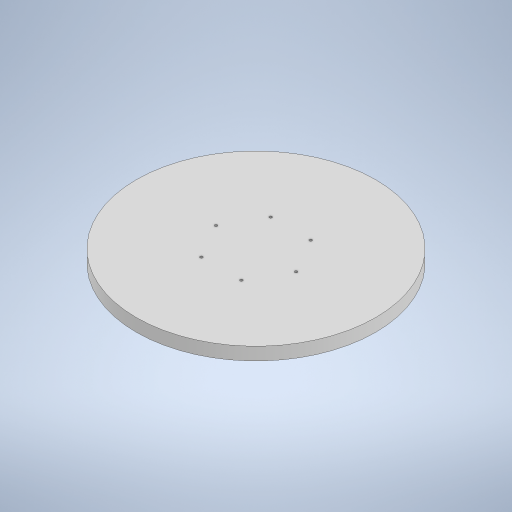
# Autodesk Inventor part: Lazy suzan Top piece
Saved by Autodesk Inventor 2023 (Build 270158000, 158)
## iProperties
Created: 2022-11-23
Part Number: Lazy suzan Top piece
Material: Generic
Document SubType Name: Modeling
Designer: surat
Density: 1 g/cm^3
Appearance: Default
Author: surat
Autodesk Inventor part; units mm, degrees
ref_plane "YZ Plane" through (0, 0, 0) normal (1, 0, 0) x (0, 1, 0)
ref_plane "XZ Plane" through (0, 0, 0) normal (0, 1, 0) x (-1, 0, 0)
ref_plane "XY Plane" through (0, 0, 0) normal (0, 0, 1) x (1, 0, 0)
sketch "Sketch1" plane through (0, 0, 0) normal (0, 1, 0) x (-1, 0, 0)
  circle A0 centre (0, 0) radius 254
  circle A1 centre (0, 0) radius 279.4
  line L0 (0, 279.4) -> (0, -279.4)
  line L1 (-279.4, 0) -> (279.4, 0)
  line L2 (197.5656, -197.5656) -> (-197.5656, 197.5656)
  line L3 (197.5656, 197.5656) -> (-197.5656, -197.5656)
  line L4 (206.5459, -188.5854) -> (-188.5854, 206.5459)
  line L5 (188.5854, -206.5459) -> (-206.5459, 188.5854)
  line L6 (188.5854, 206.5459) -> (-206.5459, -188.5854)
  line L7 (206.5459, 188.5854) -> (-188.5854, -206.5459)
  circle A2 centre (0, 0) radius 152.4
  circle A3 centre (0, 0) radius 101.6
  circle A4 centre (0, 0) radius 88.9
  circle A5 centre (0, 0) radius 139.7
  circle A6 centre (146.05, 0) radius 3.175
  circle A7 centre (73.025, 126.483) radius 3.175
  circle A8 centre (-73.025, 126.483) radius 3.175
  circle A9 centre (-146.05, 0) radius 3.175
  circle A10 centre (-73.025, -126.483) radius 3.175
  circle A11 centre (73.025, -126.483) radius 3.175
  circle A12 centre (95.25, 0) radius 3.175
  circle A13 centre (47.625, 82.4889) radius 3.175
  circle A14 centre (-47.625, 82.4889) radius 3.175
  circle A15 centre (-95.25, 0) radius 3.175
  circle A16 centre (-47.625, -82.4889) radius 3.175
  circle A17 centre (47.625, -82.4889) radius 3.175
  circle A18 centre (0, 0) radius 284.48
  dimension "d0" = 508
  dimension "d1" = 25.4
  dimension "d2" = 45
  dimension "d3" = 0
  dimension "d4" = 0
  dimension "d5" = 45
  dimension "d6" = 12.7
  dimension "d7" = 12.7
  dimension "d8" = 12.7
  dimension "d9" = 12.7
  dimension "d10" = 304.8
  dimension "d11" = 203.2
  dimension "d12" = 177.8
  dimension "d13" = 12.7
  dimension "d14" = 6.35
  dimension "d15" = 146.05
  dimension "d18" = 360
  dimension "d20" = 6.35
  dimension "d21" = 95.25
  dimension "d24" = 360
  dimension "d26" = 5.08
  constraints: 18 centre point, 16 end point, 5 coincident, 4 parallel, 2 midpoint, 2 point on line, 1 perpendicular, 1 vertical, 36 other
  measures "d0" diameter of A0
  measures "d2" angle of L3 L0
  measures "d3" distance from line of point (0, 0) L3
  measures "d4" distance from line of point (0, 0) L2
  measures "d5" angle of L0 L2
  measures "d6" distance between parallel lines of L2 L4
  measures "d7" distance between parallel lines of L2 L5
  measures "d8" distance between parallel lines of L3 L6
  measures "d9" distance between parallel lines of L3 L7
  measures "d10" diameter of A2
  measures "d11" diameter of A3
  measures "d12" diameter of A4
  measures "d13" radial gap between concentric circles of A2 A5
  measures "d14" diameter of A6
  measures "d15" distance of A5.centre A6.centre
  measures "d20" diameter of A12
  measures "d21" distance of A4.centre A12.centre
extrude "Extrusion1" add sketch "Sketch1" along normal blind 5.08 contours L1 A2 L7 A0 | L1 A1 L4 A0 | A0 L4 A2 L1 | A0 L7 A1 L1 | L7 A2 L3 A0 | A0 L3 A1 L7 | L4 A1 L2 A0 | A0 L2 A2 L4 | A2 L4 A5 L1 A6 | L1 A6 A5 L7 A2 | L3 A2 L6 A0 | A0 L6 A1 L3 | L7 A5 L3 A2 | L2 A1 L5 A0 | A0 L5 A2 L2 | A2 L2 A5 L4 | A6 L1 | L1 A6 | L6 A2 L0 A0 | A0 L0 A1 L6 | L3 A5 L6 A2 | A5 L1 A3 L7 | L7 A3 L3 A5 | L5 A1 L0 A0 | A0 L0 A2 L5 | A2 L5 A5 L2 | A5 L2 A3 L4 | L4 A3 L1 A5 | L0 A2 L4 A0 | A0 L4 A1 L0 | L6 A5 L0 A2 | L3 A3 L6 A5 | A3 L1 A12 A4 L7 | L7 A4 L3 A3 | L0 A1 L7 A0 | A0 L7 A2 L0 | A2 L0 A5 L5 | A5 L5 A3 L2 | A3 L2 A4 L4 | L4 A4 L1 A12 A3 | L4 A2 L2 A0 | A0 L2 A1 L4 | L0 A5 L4 A2 | L6 A3 L0 A5 | L3 A4 L6 A3 | A4 L1 L7 | L7 L4 L3 A4 | L7 A1 L3 A0 | A0 L3 A2 L7 | A2 L7 A5 L0 | A5 L0 A3 L5 | A3 L5 A4 L2 | A4 L2 L7 L4 | L4 L1 A4 | L2 A2 L5 A0 | A0 L5 A1 L2 | L4 A5 L2 A2 | L0 A3 L4 A5 | L6 A4 L0 A3 | L3 L4 L6 A4 | L7 L2 L1 | L1 L3 L4 | L3 A1 L6 A0 | A0 L6 A2 L3 | A2 L3 A5 L7 | A5 L7 A3 L0 | A3 L0 A4 L5 | A4 L5 L7 L2 | L5 A2 L1 A0 | A0 L1 A1 L5 | L2 A5 L5 A2 | L4 A3 L2 A5 | L0 A4 L4 A3 | L6 L0 A4 | L3 L0 L4 | L2 L6 L0 | L2 L7 L0 | L3 L5 L1 | L1 L6 L2 | L0 L5 L3 | L6 A1 L1 A0 | A0 L1 A2 L6 | A2 L6 A5 L3 | A5 L3 A3 L7 | A3 L7 A4 L0 | A4 L0 L5 | L5 A5 L1 A9 A2 | L2 A3 L5 A5 | L4 A4 L2 A3 | L0 L4 A4 | L6 L2 A4 L4 | L7 A4 L3 L5 | L0 A4 L7 | L6 A4 L1 | L1 A4 L5 | L5 A4 L2 L6 | L5 L3 A4 L6 | A2 L1 A9 A5 L6 | A5 L6 A3 L3 | A3 L3 A4 L7 | L5 A3 L1 A5 | L2 A4 L5 A3 | A4 L6 A3 L1 A15 | L1 A15 A3 L5 A4 | A4 L3 A3 L6 | A5 L1 A3 L6 | A9 L1 | L1 A9 | A7 | A8 | A10 | A11 | A18
extrude "Extrusion2" add sketch "Sketch1" against normal blind 25.4 contours A18
body "Solid1"
